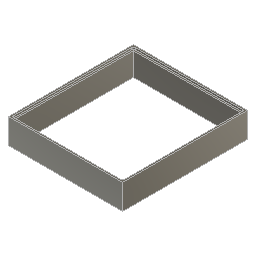
idk-what-to-call-this (Autodesk Fusion 360 design; units mm, degrees)
Autodesk Fusion 360 part; units mm, degrees
sketch "Sketch1" plane through (0, 0, 3.175) normal (0, 0, 1) x (-1, 0, 0)
  line L0 (0, 0) -> (0, 297.942)
  line L1 (0, 297.942) -> (-407.924, 297.942)
  line L2 (-407.924, 297.942) -> (-407.924, 0)
  line L3 (-407.924, 0) -> (0, 0)
  line L4 (-201.1, 0) -> (-201.1, 177.942)
  line L5 (-134.55, 148.972) -> (-201.1, 148.972)
  line L6 (-134.55, 148.972) -> (-51.1, 148.972)
  line L7 (-65, 148.972) -> (-65, 0)
  line L8 (-65, 0) -> (-201.1, 0)
  line L9 (-201.1, 0) -> (-201.1, 148.972)
  line L10 (-201.1, 148.972) -> (-65, 148.972)
  line L11 (-65, 148.972) -> (-65, 0)
  line L12 (-197.1, 144.972) -> (-69, 144.972)
  line L13 (-69, 144.972) -> (-69, 4)
  line L14 (-69, 4) -> (-197.1, 4)
  line L15 (-197.1, 4) -> (-197.1, 144.972)
  dimension "d280" = 4
  constraint horizontal L8
  constraint vertical L9
  constraint horizontal L10
  constraint vertical L11
  constraint coincident L5.end L9.end
  constraint coincident L7.end L8.start
extrude "Extrude1" add sketch "Sketch1" along normal blind 30 contours L3 L4 L5 L6 L7 L8 L9 L10 L11
sketch "Sketch2" plane through (0, 0, 33.175) normal (0, 0, 1) x (-1, 0, 0)
  line L0 (-69, 4) -> (-197.1, 4)
  line L1 (-197.1, 4) -> (-197.1, 144.972)
  line L2 (-197.1, 144.972) -> (-69, 144.972)
  line L3 (-69, 144.972) -> (-69, 4)
  line L4 (-65, 148.972) -> (-201.1, 148.972)
  line L5 (-201.1, 148.972) -> (-201.1, 0)
  line L6 (-201.1, 0) -> (-65, 0)
  line L7 (-65, 0) -> (-65, 148.972)
  line L8 (-199.1, 4) -> (-199.1, 144.972)
  line L9 (-197.1, 146.972) -> (-69, 146.972)
  line L10 (-67, 144.972) -> (-67, 4)
  line L11 (-69, 2) -> (-197.1, 2)
  arc A0 (-69, 2) -> (-67, 4) centre (-69, 4) ccw
  arc A1 (-67, 144.972) -> (-69, 146.972) centre (-69, 144.972) ccw
  arc A2 (-197.1, 146.972) -> (-199.1, 144.972) centre (-197.1, 144.972) ccw
  arc A3 (-199.1, 4) -> (-197.1, 2) centre (-197.1, 4) ccw
  dimension "d284" = 2
  constraint tangent L11 A0
  constraint tangent L10 A0
  constraint tangent L10 A1
  constraint tangent L9 A1
  constraint equal A0 A1
  constraint tangent L9 A2
  constraint tangent L8 A2
  constraint equal A0 A2
  constraint tangent L8 A3
  constraint tangent L11 A3
  constraint equal A0 A3
  measures "d284" radius of A0
extrude "Extrude2" cut sketch "Sketch2" against normal blind 2.5 contours L8 L9 L10 L11 A0 A1 A2 A3
equation "d280 = ComponentWallWidth"
equation "ComponentWallWidth = 4 mm"
